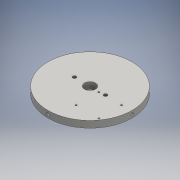
# Autodesk Inventor part: outsideCover
Saved by Autodesk Inventor 2016 (Build 200138000, 138)
## iProperties
Created: 2016-10-27
Part Number: outsideCover
Material: 一般
Document SubType Name: Modeling
Designer: Daisuke
Density: 1 g/cm^3
Appearance: 既定
Author: Daisuke
Autodesk Inventor part; units mm, degrees
ref_plane "XY Plane" through (0, 0, 0) normal (0, 0, 1) x (1, 0, 0)
sketch "スケッチ1" plane through (0, 0, 0) normal (0, 0, 1) x (1, 0, 0)
  circle A0 centre (0, 0) radius 50
  dimension "d0" = 100
  constraints: 1 centre point, 1 coincident
  measures "d0" diameter of A0
extrude "押し出し1" add sketch "スケッチ1" along normal blind 8
ref_plane "作業平面1" through (50, 0, 0) normal (1, 0, 0) x (0, 1, 0)
ref_plane "作業平面2" through (-50, 0, 0) normal (1, 0, 0) x (0, 1, 0)
ref_plane "作業平面3" through (0, 50, 0) normal (0, 1, 0) x (-1, 0, 0)
ref_plane "作業平面4" through (0, -50, 0) normal (0, 1, 0) x (-1, 0, 0)
sketch "スケッチ2" plane through (50, 0, 0) normal (1, 0, 0) x (0, 1, 0)
  line L0 (0, 0) -> (0, 4) construction
  circle A0 centre (0, 4) radius 1.5
  dimension "d7" = 4
  dimension "d8" = 3
  constraints: 2 end point, 1 centre point, 1 coincident, 1 vertical
  measures "d7" distance of L0.start L0.end
  measures "d8" diameter of A0
extrude "押し出し2" cut sketch "スケッチ2" against normal blind 5
sketch "スケッチ3" plane through (-50, 0, 0) normal (1, 0, 0) x (0, 1, 0)
  line L0 (0, 0) -> (0, 4) construction
  circle A0 centre (0, 4) radius 1.5
  dimension "d11" = 4
  dimension "d12" = 3
  constraints: 2 end point, 1 centre point, 1 coincident, 1 vertical
  measures "d11" distance of L0.start L0.end
  measures "d12" diameter of A0
extrude "押し出し3" cut sketch "スケッチ3" along normal blind 5
sketch "スケッチ4" plane through (0, 50, 0) normal (0, 1, 0) x (-1, 0, 0)
  line L0 (0, 0) -> (0, 4) construction
  circle A0 centre (0, 4) radius 1.5
  dimension "d15" = 4
  dimension "d16" = 3
  constraints: 2 end point, 1 centre point, 1 coincident, 1 vertical
  measures "d15" distance of L0.start L0.end
  measures "d16" diameter of A0
extrude "押し出し4" cut sketch "スケッチ4" against normal blind 5
sketch "スケッチ5" plane through (0, -50, 0) normal (0, 1, 0) x (-1, 0, 0)
  line L0 (0, 0) -> (0, 4) construction
  circle A0 centre (0, 4) radius 1.5
  dimension "d19" = 4
  dimension "d20" = 3
  constraints: 2 end point, 1 centre point, 1 coincident, 1 vertical
  measures "d19" distance of L0.start L0.end
  measures "d20" diameter of A0
extrude "押し出し5" cut sketch "スケッチ5" along normal blind 5
thread "ねじ1" size "M3x0.5" class "6H" standard "ANSI Metric M Profile" full length
thread "ねじ2" size "M3x0.5" class "6H" standard "ANSI Metric M Profile" full length
thread "ねじ3" size "M3x0.5" class "6H" standard "ANSI Metric M Profile" full length
thread "ねじ4" size "M3x0.5" class "6H" standard "ANSI Metric M Profile" full length
sketch "スケッチ6" plane through (0, 0, 8) normal (0, 0, 1) x (1, 0, 0)
  line L0 (25, -25) -> (25, 0) construction
  line L1 (25, -9.5) -> (25, 0) construction
  circle A0 centre (11.5, -1) radius 1
  circle A1 centre (38.5, -1) radius 1
  line L2 (25, -9.5) -> (25, -28) construction
  circle A2 centre (11.5, -28) radius 1
  circle A3 centre (38.5, -28) radius 1
  line L3 (11.5, -28) -> (25, -28) construction
  line L4 (4.7131, -23.5519) -> (5.4895, -20.6541) construction
  line L5 (38.5, -1) -> (38.5, -25) construction
  line L6 (38.5, -1) -> (25, -1) construction
  circle A4 centre (0, -0.0236) radius 6 construction
  circle A5 centre (0, -0.0236) radius 15 construction
  circle A6 centre (25.2091, -0.0236) radius 10 construction
  circle A7 centre (25.2091, -0.0236) radius 3 construction
  line L7 (0, -0.0236) -> (50, -0.0236) construction
  circle A8 centre (0, 0) radius 50 construction
  line L8 (0, -0.0236) -> (0, -50) construction
  circle A9 centre (25.2091, -0.0236) radius 13.5 construction
  line L9 (11.7091, -0.0236) -> (11.7091, 1.9764) construction
  line L10 (11.7091, 1.9764) -> (11.858, 1.9764) construction
  point P0 (25, -25)
  point P1 (25, -25)
  dimension "d43" = 25
  dimension "d46" = 2
  dimension "d48" = 2
  dimension "d50" = 2
  dimension "d51" = 2
  dimension "d53" = 13.5
  dimension "d54" = 3
  dimension "d55" = 24
  dimension "d56" = 13.5
  dimension "d69" = 12
  dimension "d70" = 30
  dimension "d71" = 20
  dimension "d72" = 6
  dimension "d77" = 27
  dimension "d78" = 2
  constraints: 22 end point, 9 centre point, 4 point on circle, 3 coincident, 2 horizontal, 2 point on line, 1 perpendicular, 1 tangent
  measures "d43" distance of L0.start L0.end
  measures "d46" diameter of A0
  measures "d48" diameter of A1
  measures "d50" diameter of A2
  measures "d51" diameter of A3
  measures "d53" distance of L3.start L2.end
  measures "d54" distance of L4.start L4.end
  measures "d55" distance of L5.start L5.end
  measures "d56" distance of L5.start L6.end
  measures "d69" diameter of A4
  measures "d70" diameter of A5
  measures "d71" diameter of A6
  measures "d72" diameter of A7
  measures "d77" diameter of A9
  measures "d78" distance of L9.start L9.end
extrude "押し出し6" cut sketch "スケッチ6" against normal blind 8
sketch "スケッチ8" plane through (0, 0, 8) normal (0, 0, 1) x (1, 0, 0)
  line L0 (0, 0) -> (18.5, 0) construction
  line L1 (0, 0) -> (-18.5, 0) construction
  circle A0 centre (18.5, 0) radius 2
  circle A1 centre (-18.5, 0) radius 2
  circle A2 centre (0, 0) radius 6.5
  dimension "d62" = 18.5
  dimension "d63" = 18.5
  dimension "d64" = 4
  dimension "d65" = 4
  dimension "d66" = 13
  constraints: 4 end point, 3 centre point, 3 coincident, 2 horizontal
  measures "d62" distance of L0.start L0.end
  measures "d63" distance of L0.start L1.end
  measures "d64" diameter of A0
  measures "d65" diameter of A1
  measures "d66" diameter of A2
extrude "押し出し7" cut sketch "スケッチ8" against normal blind 8
thread "ねじ7" size "M4x0.7" class "6H" standard "ANSI Metric M Profile" full length
thread "ねじ8" size "M4x0.7" class "6H" standard "ANSI Metric M Profile" full length
